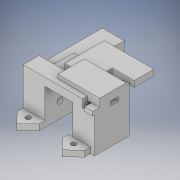
# Autodesk Inventor part: game-over
Saved by Autodesk Inventor 2017 (Build 210142000, 142)
## iProperties
Created: 2017-03-05
Part Number: game-over
Material: Generic
Document SubType Name: Modeling
Designer: John
Density: 1 g/cm^3
Appearance: Default
Author: John
Autodesk Inventor part; units mm, degrees
ref_plane "YZ Plane" through (0, 0, 0) normal (1, 0, 0) x (0, 1, 0)
ref_plane "XY Plane" through (0, 0, 0) normal (0, 0, 1) x (1, 0, 0)
sketch "Sketch1" plane through (0, 0, 0) normal (0, 1, 0) x (-1, 0, 0)
  line L0 (0, 0) -> (80, 0) construction
  line L1 (80, 0) -> (80, 15) construction
  line L2 (80, 15) -> (0, 15) construction
  line L3 (0, 15) -> (0, 0) construction
  dimension "d0" = 80
  dimension "d1" = 15
  constraints: 8 end point, 2 parallel, 1 horizontal, 1 perpendicular
  measures "d0" distance of L2.end L1.end
  measures "d1" distance of L1.end L0.end
sketch "Sketch2" plane through (0, 0, 0) normal (0, 1, 0) x (-1, 0, 0)
  line L0 (80, -20) -> (69, -20)
  line L1 (69, -20) -> (69, 20)
  line L2 (69, 20) -> (80, 20)
  line L3 (80, 20) -> (80, -20)
  line L4 (55, 0) -> (44, 0)
  line L5 (44, 0) -> (44, 20)
  line L6 (44, 20) -> (55, 20)
  line L7 (55, 20) -> (55, 0)
  line L8 (71, -18) -> (78, -18)
  line L9 (78, -18) -> (78, 18)
  line L10 (78, 18) -> (71, 18)
  line L11 (71, 18) -> (71, -18)
  line L12 (53, 2) -> (46, 2)
  line L13 (46, 2) -> (46, 18)
  line L14 (46, 18) -> (53, 18)
  line L15 (53, 18) -> (53, 2)
  dimension "d2" = 11
  dimension "d3" = 40
  dimension "d6" = 11
  dimension "d10" = 2
  dimension "d11" = 2
  dimension "d110" = 20
  dimension "d111" = 14
  constraints: 32 end point, 8 parallel, 4 perpendicular, 2 horizontal, 1 collinear, 6 other
  measures "d2" distance of L1.end L2.end
  measures "d3" distance of L0.end L1.end
  measures "d6" distance of L5.end L6.end
  measures "d10" distance between parallel lines of L0 L8
  measures "d11" distance between parallel lines of L7 L15
  measures "d110" distance of L6.end L4.start
  measures "d111" distance between parallel lines of L7 L1
extrude "Extrusion1" add sketch "Sketch2" along normal blind 15
sketch "Sketch3" plane through (0, 15, 0) normal (0, 1, 0) x (1, 0, 0)
  line L0 (-69, 20) -> (-80, 20) projected
  line L1 (-80, 20) -> (-69, 20)
  line L2 (-69, 20) -> (-69, -20)
  line L3 (-69, -20) -> (-80, -20)
  line L4 (-80, -20) -> (-80, 20)
  line L5 (-55, -20) -> (-44, -20) projected
  line L6 (-44, -20) -> (-55, -20)
  line L7 (-55, -20) -> (-55, 0)
  line L8 (-55, 0) -> (-44, 0)
  line L9 (-44, 0) -> (-44, -20)
  point P0 (0, 0)
  dimension "d16" = 40
  constraints: 16 end point, 4 parallel, 2 horizontal, 2 perpendicular
  measures "d16" distance of L1.end L2.end
extrude "Extrusion2" add sketch "Sketch3" along normal blind 3
sketch "Sketch4" plane through (-69, 0, 20) normal (1, 0, 0) x (0, 0, -1)
  circle A0 centre (7.5, 8) radius 1.5
  line L0 (2, 0) -> (38, 0) projected
  line L1 (0, 0) -> (0, 18) construction
  point P0 (0, 15)
  dimension "d26" = 3
  dimension "d28" = 8
  dimension "d29" = 7.5
  constraints: 1 centre point
  measures "d26" diameter of A0
  measures "d28" distance from line of L0 A0.centre
  measures "d29" distance from line of L1 A0.centre
extrude "Extrusion3" cut sketch "Sketch4" against normal blind 3
sketch "Sketch5" plane through (-55, 0, 0) normal (-1, 0, 0) x (0, 0, 1)
  circle A0 centre (12.5, 8) radius 1.5
  line L0 (20, 0) -> (20, 18) projected
  line L1 (2, 0) -> (18, 0) projected
  point P0 (0, 0)
  point P1 (20, 15)
  dimension "d33" = 3
  dimension "d34" = 7.5
  dimension "d35" = 8
  constraints: 1 centre point
  measures "d33" diameter of A0
  measures "d34" distance from line of L0 A0.centre
  measures "d35" distance from line of L1 A0.centre
extrude "Extrusion4" cut sketch "Sketch5" against normal blind 3
ref_plane "Work Plane1" through (0, 18, 0) normal (0, 1, 0) x (-1, 0, 0)
sketch "Sketch12" plane through (0, 18, 0) normal (0, 1, 0) x (-1, 0, 0)
  line L0 (80, 20) -> (50, 20)
  line L1 (50, 20) -> (50, 12)
  line L2 (50, 12) -> (80, 12)
  line L3 (80, 12) -> (80, 20)
  line L4 (55, 0) -> (25, 0)
  line L5 (25, 0) -> (25, 8)
  line L6 (25, 8) -> (55, 8)
  line L7 (55, 8) -> (55, 0)
  line L8 (32, 2) -> (32, 18) projected
  line L9 (32, 12) -> (2, 12)
  line L10 (2, 12) -> (2, 20)
  line L11 (2, 20) -> (32, 20)
  line L12 (32, 20) -> (32, 12)
  point P0 (0, 0)
  dimension "d59" = 30
  dimension "d60" = 8
  dimension "d61" = 30
  dimension "d62" = 8
  dimension "d63" = 30
  constraints: 24 end point, 6 parallel, 3 horizontal, 3 perpendicular, 3 point on line
  measures "d59" distance of L2.end L1.end
  measures "d60" distance of L1.end L0.end
  measures "d61" distance of L5.end L6.end
  measures "d62" distance of L4.end L5.end
  measures "d63" distance of L10.end L11.end
sketch "Sketch13" plane through (0, 18, 0) normal (0, 1, 0) x (-1, 0, 0)
  line L0 (74.3573, 0) -> (62.3573, 0)
  line L1 (62.3573, 0) -> (62.3573, 15)
  line L2 (62.3573, 15) -> (74.3573, 15)
  line L3 (74.3573, 15) -> (74.3573, 0)
  line L4 (48, 12) -> (36, 12)
  line L5 (36, 12) -> (36, 21)
  line L6 (36, 21) -> (48, 21)
  line L7 (48, 21) -> (48, 12)
  line L8 (0, 0) -> (11, 0) projected
  line L9 (4, 0) -> (17, 0)
  line L10 (17, 0) -> (17, 17)
  line L11 (17, 17) -> (4, 17)
  line L12 (4, 17) -> (4, 0)
  dimension "d64" = 12
  dimension "d65" = 15
  dimension "d66" = 12
  dimension "d67" = 13
  dimension "d68" = 17
  constraints: 24 end point, 6 parallel, 3 horizontal, 3 perpendicular, 1 point on line
  measures "d64" distance of L1.end L2.end
  measures "d65" distance of L0.end L1.end
  measures "d66" distance of L5.end L6.end
  measures "d67" distance of L11.end L10.end
  measures "d68" distance of L10.end L9.end
extrude "Extrusion9" add sketch "Sketch13" along normal blind 2
extrude "Extrusion10" add sketch "Sketch12" along normal blind 4
sketch "Sketch14" plane through (0, 20, 0) normal (0, 1, 0) x (1, 0, 0)
  line L0 (-65, -4) -> (-41.7529, -4)
  line L1 (-41.7529, -4) -> (-41.7529, -17.4715)
  line L2 (-41.7529, -17.4715) -> (-65, -17.4715)
  line L3 (-65, -17.4715) -> (-65, -4)
  point P0 (0, 0)
  constraints: 8 end point, 2 parallel, 1 horizontal, 1 perpendicular
extrude "Extrusion11" add sketch "Sketch14" along normal blind 4
sketch "Sketch15" plane through (0, 20, 0) normal (0, 1, 0) x (1, 0, 0)
  line L0 (-69, -15) -> (-69, 0) projected
  line L1 (-69, -10) -> (-17, -10)
  line L2 (-17, -10) -> (-17, 10)
  line L3 (-17, 10) -> (-69, 10)
  line L4 (-69, 10) -> (-69, -10)
  point P0 (0, 0)
  point P1 (-69, -20)
  point P2 (-69, -22)
  point P3 (-69, -20)
  dimension "d76" = 52
  dimension "d77" = 20
  constraints: 8 end point, 2 parallel, 1 horizontal, 1 perpendicular, 1 point on line
  measures "d76" distance of L3.end L2.end
  measures "d77" distance of L2.end L1.end
extrude "Extrusion12" add sketch "Sketch15" along normal blind 3
sketch "Sketch16" plane through (0, 0, 0) normal (0, 1, 0) x (-1, 0, 0)
  line L0 (69, 20) -> (80, 20) projected
  line L1 (80, 20) -> (80, 23)
  line L2 (69, 20) -> (69, 23)
  line L3 (69, 23) -> (74.8182, 28.4908)
  line L4 (74.8182, 28.4908) -> (80, 23)
  circle A0 centre (74.5, 23) radius 1.25
  line L5 (74.5, 23) -> (80, 23) construction
  line L6 (74.5, 23) -> (69, 23) construction
  line L7 (80, 15) -> (0, 15) construction
  line L8 (46, 20) -> (46, 23)
  line L9 (51.5, 23) -> (46, 23) construction
  circle A1 centre (51.5, 23) radius 1.25
  line L10 (57, 20) -> (57, 23)
  line L11 (51.5, 23) -> (57, 23) construction
  line L12 (51.8182, 28.4908) -> (57, 23)
  line L13 (46, 23) -> (51.8182, 28.4908)
  line L14 (57, 20) -> (46, 20)
  dimension "d80" = 3
  dimension "d81" = 3
  dimension "d82" = 8
  dimension "d83" = 2.5
  dimension "d84" = 3
  dimension "d96" = 23
  constraints: 28 end point, 2 centre point, 2 collinear, 2 horizontal, 2 vertical, 1 perpendicular, 12 other
  measures "d80" distance of L0.end L1.end
  measures "d81" distance of L0.start L2.end
  measures "d82" distance of L2.end L3.end
  measures "d83" diameter of A0
  measures "d84" distance from line of L0 L5.start
  measures "d96" distance of L0.start L8.start
extrude "Extrusion14" add sketch "Sketch16" along normal blind 3
sketch "Sketch17" plane through (0, 0, 0) normal (0, 1, 0) x (-1, 0, 0)
  line L0 (44, 21.1125) -> (0, 21.1125)
  line L1 (0, 21.1125) -> (0, -22.6665)
  line L2 (0, -22.6665) -> (44, -22.6665)
  line L3 (44, -22.6665) -> (44, 21.1125)
  line L4 (44, 0) -> (44, 20) projected
  constraints: 8 end point, 2 parallel, 1 collinear, 1 horizontal, 1 perpendicular
extrude "Extrusion15" cut sketch "Sketch17" along normal through all
sketch "Sketch18" plane through (0, 0, 0) normal (0, 1, 0) x (-1, 0, 0)
  line L0 (26.5385, 0) -> (55, 4)
  line L1 (55, 4) -> (55, 0)
  line L2 (55, 0) -> (26.5385, 0)
  line L3 (55, 23) -> (55, 20) projected
  line L4 (55, 0) -> (44, 0) projected
  line L5 (69, -20) -> (69, 23) projected
  point P0 (0, 0)
  point P1 (57, 23)
  point P2 (57, 20)
  point P3 (69, 20)
  dimension "d103" = 8
  dimension "d104" = 4
  constraints: 6 end point, 2 vertical, 1 collinear, 1 perpendicular, 1 other
  measures "d103" angle of L2 L0
  measures "d104" distance of L0.end L1.end
extrude "Extrusion16" cut sketch "Sketch18" along normal through all
equation "\"d11\" = d10"
equation "\"d81\" = d80"
equation "\"d84\" = d81"
body "Solid1"
